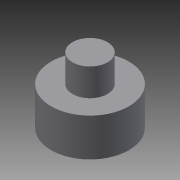
# Autodesk Inventor part: hridel kuzelova kolecka
Saved by Autodesk Inventor 2015 (Build 190159000, 159)
## iProperties
Created: 2012-08-16
Part Number: hridel kuzelova kolecka
Material: Generic
Document SubType Name: Modeling
Designer: idle-rug
Density: 1 g/cm^3
Appearance: Default
Author: idle-rug
Autodesk Inventor part; units mm, degrees
ref_plane "YZ Plane" through (0, 0, 0) normal (1, 0, 0) x (0, 1, 0)
ref_plane "XZ Plane" through (0, 0, 0) normal (0, 1, 0) x (-1, 0, 0)
ref_plane "XY Plane" through (0, 0, 0) normal (0, 0, 1) x (1, 0, 0)
sketch "Sketch1" plane through (0, 0, 0) normal (0, 0, 1) x (1, 0, 0)
  circle A0 centre (0, 0) radius 6.65
  dimension "d0" = 13.3
  constraints: 1 centre point, 1 coincident
  measures "d0" diameter of A0
extrude "Extrusion1" add sketch "Sketch1" along normal blind 6.5
ref_plane "Work Plane1" through (-6.65, 6.65, 6.5) normal (0, 1, 0) x (1, 0, 0)
sketch "Sketch3" plane through (-6.65, 6.65, 6.5) normal (0, 1, 0) x (1, 0, 0)
  circle A0 centre (6.65, 3.25) radius 1.2
  dimension "d9" = 2.4
  constraints: 1 centre point
  measures "d9" diameter of A0
hole "Hole1" at (0, 6.65, 3.25) direction (0, -1, 0) diameter 2.459 depth 6.65 thread size "M3x0.5" designation "M3" class "6H" standard "GB Metric profile"
sketch "Sketch4" plane through (0, 0, 6.5) normal (0, 0, 1) x (1, 0, 0)
  circle A0 centre (0, 0) radius 6.65 projected
  circle A1 centre (0, 0) radius 3
  dimension "d17" = 6
  constraints: 1 centre point, 1 coincident
  measures "d17" diameter of A1
extrude "Extrusion3" add sketch "Sketch4" along normal blind 4.7 contours A1
body "Solid1"
